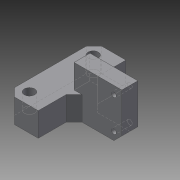
# Autodesk Inventor part: Col support top
Saved by Autodesk Inventor 2015 (Build 190159000, 159)
## iProperties
Created: 2019-01-12
Part Number: Col support top
Material: Generic
Document SubType Name: Modeling
Designer: Toby
Density: 1 g/cm^3
Appearance: Default
Author: Toby
Autodesk Inventor part; units mm, degrees
ref_plane "YZ Plane" through (0, 0, 0) normal (1, 0, 0) x (0, 1, 0)
ref_plane "XZ Plane" through (0, 0, 0) normal (0, 1, 0) x (-1, 0, 0)
ref_plane "XY Plane" through (0, 0, 0) normal (0, 0, 1) x (1, 0, 0)
sketch "Sketch1" plane through (0, 0, 0) normal (0, 0, 1) x (1, 0, 0)
  line L0 (-5.4307, 20.6828) -> (14.5693, 20.6828)
  line L1 (14.5693, 20.6828) -> (14.5693, -34.3172)
  line L2 (14.5693, -34.3172) -> (-5.4307, -34.3172)
  line L3 (-5.4307, -34.3172) -> (-5.4307, 20.6828)
  point P0 (0, 0)
  dimension "d0" = 55
  dimension "d1" = 20
  constraints: 8 end point, 2 parallel, 1 horizontal, 1 perpendicular
  measures "d0" distance of L2.end L0.start
  measures "d1" distance of L0.start L0.end
extrude "Extrusion1" add sketch "Sketch1" along normal blind 15
sketch "Sketch2" plane through (0, 0, 15) normal (0, 0, 1) x (1, 0, 0)
  line L0 (14.5693, 20.6828) -> (-5.4307, 20.6828) projected
  line L1 (-5.4307, -34.3172) -> (-5.4307, 20.6828) projected
  line L2 (-5.4307, -34.3172) -> (14.5693, -34.3172) projected
  circle A0 centre (1.5693, 13.1828) radius 3.25
  circle A1 centre (1.5693, -26.8172) radius 3.25
  point P0 (0, 0)
  dimension "d4" = 40
  dimension "d5" = 7.5
  dimension "d6" = 7
  dimension "d7" = 7.5
  dimension "d8" = 6.5
  dimension "d9" = 6.5
  constraints: 2 centre point, 2 coincident
  measures "d4" distance of point (1.569, -26.817) point (1.569, 13.183)
  measures "d5" distance from line of L0 point (1.569, 13.183)
  measures "d6" distance from line of L1 point (1.569, 13.183)
  measures "d7" distance from line of L2 point (1.569, -26.817)
  measures "d8" diameter of A0
  measures "d9" diameter of A1
extrude "Extrusion2" cut sketch "Sketch2" against normal blind 10
sketch "Sketch3" plane through (0, 0, 0) normal (0, 0, -1) x (-1, 0, 0)
  line L0 (-14.5693, -34.3172) -> (-14.5693, 20.6828) projected
  line L1 (-14.5693, -1.8172) -> (-44.5693, -1.8172)
  line L2 (-44.5693, -1.8172) -> (-44.5693, -11.8172)
  line L3 (-44.5693, -11.8172) -> (-14.5693, -11.8172)
  line L4 (-14.5693, -11.8172) -> (-14.5693, -1.8172)
  line L5 (5.4307, 20.6828) -> (5.4307, -34.3172) projected
  point P0 (0, 0)
  point P1 (5.4307, -6.8172)
  dimension "d12" = 10
  dimension "d13" = 5
  dimension "d14" = 30
  constraints: 8 end point, 2 parallel, 1 horizontal, 1 midpoint, 1 perpendicular, 1 point on line
  measures "d12" distance between parallel lines of L3 L1
  measures "d13" distance from line of point (5.431, -6.817) L1
  measures "d14" distance between parallel lines of L0 L2
extrude "Extrusion3" add sketch "Sketch3" against normal blind 30
sketch "Sketch4" plane through (14.5693, -1.8172, 0) normal (0, 1, 0) x (1, 0, 0)
  line L0 (30, 0) -> (0, 0) projected
  line L1 (30, 0) -> (30, -30) projected
  line L2 (30, -30) -> (0, -30) projected
  point P0 (-14.5693, 0)
  point P1 (25, -5)
  point P2 (25, -25)
  dimension "d17" = 5
  dimension "d18" = 5
  dimension "d19" = 5
  dimension "d20" = 5
  measures "d17" distance from line of L0 point (25, -5)
  measures "d18" distance from line of L1 point (25, -5)
  measures "d19" distance from line of L1 point (25, -25)
  measures "d20" distance from line of L2 point (25, -25)
hole "Hole1" at (39.5693, -1.8172, 5) at (39.5693, -1.8172, 25) direction (0, -1, 0) diameter 3 depth 10 tip angle 118
chamfer "Chamfer1" distance 5 angle 45 1 edges at (44.5693, -6.8172, 0)
chamfer "Chamfer2" distance 5 angle 45 2 edges at (14.5693, -1.8172, 7.5) (14.5693, -11.8172, 7.5)
chamfer "Chamfer3" distance 5 angle 45 2 edges at (-5.4307, -34.3172, 7.5) (-5.4307, 20.6828, 7.5)
body "Solid1"
